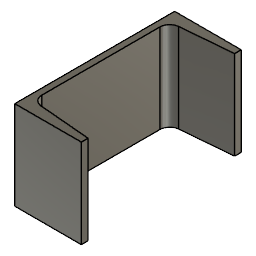
C-180×75×7×10.5 (Autodesk Fusion 360 design; units mm, degrees)
Autodesk Fusion 360 part; units mm, degrees
note: some values were not read from the file. Set by a fixed rule: which sketch regions a step uses.
sketch "スケッチ1" plane through (0, 0, 0) normal (0, 0, 1) x (1, 0, 0)
  line L0 (7, 156.4457) -> (7, 23.5543)
  line L1 (0, 180) -> (0, 0)
  line L2 (0, 0) -> (75, 0)
  line L3 (17.0413, 12.5961) -> (75, 7.5254)
  arc A0 (7, 23.5543) -> (17.0413, 12.5961) centre (18, 23.5543) ccw
  line L4 (75, 7.5254) -> (75, 0)
  line L5 (75, 172.4746) -> (17.0413, 167.4039)
  arc A1 (17.0413, 167.4039) -> (7, 156.4457) centre (18, 156.4457) ccw
  line L6 (0, 180) -> (75, 180)
  line L7 (75, 180) -> (75, 172.4746)
extrude "押し出し1" add sketch "スケッチ1" along normal blind 100
